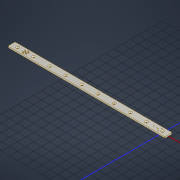
# Autodesk Inventor part: Y Extrusion-Backer [A] (350mm)
Saved by Autodesk Inventor 2022.2 (Build 262287010, 287A)
## iProperties
Created: 2022-03-23
Part Number: Y Extrusion-Backer [A] (350mm)
Material: Titan
Document SubType Name: Modeling
Designer: sleib
Density: 4.51 g/cm^3
Appearance: Titan
Author: sleib
Autodesk Inventor part; units mm, degrees
ref_plane "YZ Plane" through (0, 0, 0) normal (1, 0, 0) x (0, 1, 0)
ref_plane "XZ Plane" through (0, 0, 0) normal (0, 1, 0) x (-1, 0, 0)
ref_plane "XY Plane" through (0, 0, 0) normal (0, 0, 1) x (1, 0, 0)
sketch "ExtrusionBacker_Y_350mm_A" plane through (0, 0, 0) normal (0, 0, 1) x (1, 0, 0)
  circle A0 centre (-11.0001, 28.106) radius 1
  circle A1 centre (-11.0001, 38.106) radius 1
  arc A2 (355.9999, 24.106) -> (357.9999, 26.106) centre (355.9999, 26.106) ccw
  line L0 (357.9999, 26.106) -> (357.9999, 40.106)
  arc A3 (357.9999, 40.106) -> (355.9999, 42.106) centre (355.9999, 40.106) ccw
  line L1 (355.9999, 42.106) -> (-30.0001, 42.106)
  arc A4 (-30.0001, 42.106) -> (-32.0001, 40.106) centre (-30.0001, 40.106) ccw
  line L2 (-32.0001, 40.106) -> (-32.0001, 26.106)
  arc A5 (-32.0001, 26.106) -> (-30.0001, 24.106) centre (-30.0001, 26.106) ccw
  line L3 (-30.0001, 24.106) -> (355.9999, 24.106)
  line L4 (322.9999, 37.0031) -> (328.736, 33.6914)
  line L5 (328.736, 33.6914) -> (328.736, 36.2894)
  line L6 (328.736, 36.2894) -> (322.9999, 39.6012)
  line L7 (322.9999, 39.6012) -> (322.9999, 37.0031)
  line L8 (317.2637, 35.1187) -> (317.2637, 37.7168)
  line L9 (317.2637, 37.7168) -> (328.736, 31.0933)
  line L10 (328.736, 31.0933) -> (328.736, 28.4952)
  line L11 (328.736, 28.4952) -> (317.2637, 35.1187)
  line L12 (317.2637, 32.5207) -> (317.2637, 29.9226)
  line L13 (317.2637, 29.9226) -> (322.9999, 26.6108)
  line L14 (322.9999, 26.6108) -> (322.9999, 29.2089)
  line L15 (322.9999, 29.2089) -> (317.2637, 32.5207)
  circle A6 centre (102.9999, 33.106) radius 1.7
  circle A7 centre (142.9999, 33.106) radius 1.7
  circle A8 centre (222.9999, 33.106) radius 1.7
  circle A9 centre (182.9999, 33.106) radius 1.7
  circle A10 centre (62.9999, 33.106) radius 1.7
  circle A11 centre (302.9999, 33.106) radius 1.7
  circle A12 centre (-3.0001, 33.106) radius 1
  circle A13 centre (342.9999, 33.106) radius 1.7
  circle A14 centre (4.9999, 33.106) radius 1
  circle A15 centre (-17.0001, 33.106) radius 1.7
  circle A16 centre (22.9999, 33.106) radius 1.7
  circle A17 centre (262.9999, 33.106) radius 1.7
  circle A18 centre (-7.0001, 33.106) radius 1
sketch "Skizze1" plane through (0, 0, 0) normal (0, 1, 0) x (-1, 0, 0)
  circle A0 centre (6, -5) radius 1
  circle A1 centre (6, 5) radius 1
  arc A2 (373, -9) -> (375, -7) centre (373, -7) ccw
  line L0 (375, -7) -> (375, 7)
  arc A3 (375, 7) -> (373, 9) centre (373, 7) ccw
  line L1 (373, 9) -> (-13, 9)
  arc A4 (-13, 9) -> (-15, 7) centre (-13, 7) ccw
  line L2 (-15, 7) -> (-15, -7)
  arc A5 (-15, -7) -> (-13, -9) centre (-13, -7) ccw
  line L3 (-13, -9) -> (373, -9)
  line L4 (340, 3.8971) -> (345.7362, 0.5853)
  line L5 (345.7362, 0.5853) -> (345.7362, 3.1834)
  line L6 (345.7362, 3.1834) -> (340, 6.4952)
  line L7 (340, 6.4952) -> (340, 3.8971)
  line L8 (334.2638, 2.0127) -> (334.2638, 4.6108)
  line L9 (334.2638, 4.6108) -> (345.7362, -2.0127)
  line L10 (345.7362, -2.0127) -> (345.7362, -4.6108)
  line L11 (345.7362, -4.6108) -> (334.2638, 2.0127)
  line L12 (334.2638, -0.5853) -> (334.2638, -3.1834)
  line L13 (334.2638, -3.1834) -> (340, -6.4952)
  line L14 (340, -6.4952) -> (340, -3.8971)
  line L15 (340, -3.8971) -> (334.2638, -0.5853)
  circle A6 centre (120, 0) radius 1.7
  circle A7 centre (160, 0) radius 1.7
  circle A8 centre (240, 0) radius 1.7
  circle A9 centre (200, 0) radius 1.7
  circle A10 centre (80, 0) radius 1.7
  circle A11 centre (320, 0) radius 1.7
  circle A12 centre (14, 0) radius 1
  circle A13 centre (360, 0) radius 1.7
  circle A14 centre (22, 0) radius 1
  circle A15 centre (0, 0) radius 1.7
  circle A16 centre (40, 0) radius 1.7
  circle A17 centre (280, 0) radius 1.7
  circle A18 centre (10, 0) radius 1
  point P0 (373, -9)
  point P1 (375, 7)
  point P2 (373, 9)
  point P3 (-13, 9)
  point P4 (-15, 7)
  point P5 (-15, -7)
  point P6 (-13, -9)
  point P7 (334.2638, 2.0127)
  point P8 (334.2638, 4.6108)
  point P9 (345.7362, -2.0127)
  point P10 (345.7362, -4.6108)
  point P11 (340, 3.8971)
  point P12 (340, 6.4952)
  point P13 (345.7362, 0.5853)
  point P14 (340, -3.8971)
  point P15 (340, -6.4952)
  point P16 (334.2638, -3.1834)
  point P17 (334.2638, -0.5853)
  constraints: 1 other
extrude "Extrusion1" add sketch "Skizze1" along normal blind 3
sketch "Skizze2" plane through (0, 3, 0) normal (0, 1, 0) x (1, 0, 0)
  circle A0 centre (-360, 0) radius 1.7 projected
  circle A1 centre (-320, 0) radius 1.7 projected
  circle A2 centre (-280, 0) radius 1.7 projected
  circle A3 centre (-240, 0) radius 1.7 projected
  circle A4 centre (-200, 0) radius 1.7 projected
  circle A5 centre (-160, 0) radius 1.7 projected
  circle A6 centre (-120, 0) radius 1.7 projected
  circle A7 centre (-80, 0) radius 1.7 projected
  circle A8 centre (-40, 0) radius 1.7 projected
  circle A9 centre (0, 0) radius 1.7 projected
  constraints: 10 coincident
hole "Bohrung1" at (-360, 3, 0) at (-320, 3, 0) at (-280, 3, 0) at (-240, 3, 0) at (-200, 3, 0) at (-160, 3, 0) at (-120, 3, 0) at (-80, 3, 0) at (-40, 3, 0) at (0, 3, 0) direction (0, -1, 0) diameter 3.4 end through all countersink diameter 7.5 countersink angle 90 clearance for "Innensechskant-Senkkopfschraube DIN EN ISO 10642" size "M3" standard "DIN"
